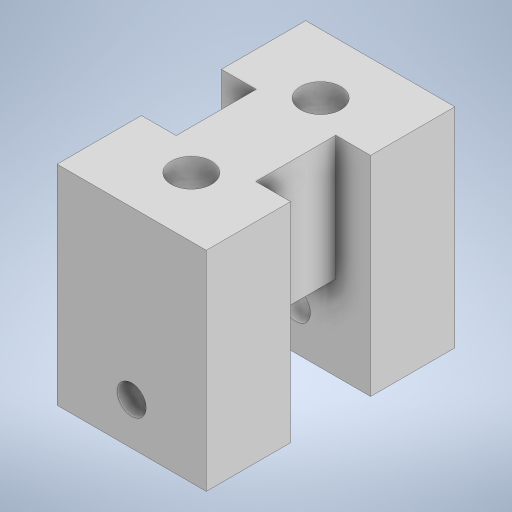
# Autodesk Inventor part: Pièce2
Saved by Autodesk Inventor 2024.1 (Build 281209000, 209)
## iProperties
Created: 2024-04-05
Part Number: Pièce2
Material: Générique
Document SubType Name: Modeling
Designer: chass
Density: 1 g/cm^3
Appearance: Par défaut
Author: chass
Autodesk Inventor part; units mm, degrees
ref_plane "YZ Plane" through (0, 0, 0) normal (1, 0, 0) x (0, 1, 0)
ref_plane "XZ Plane" through (0, 0, 0) normal (0, 1, 0) x (-1, 0, 0)
ref_plane "XY Plane" through (0, 0, 0) normal (0, 0, 1) x (1, 0, 0)
sketch "Esquisse1" plane through (0, 0, 0) normal (0, 1, 0) x (-1, 0, 0)
  line L0 (15, 25) -> (-15, 25)
  line L1 (-15, 25) -> (-15, -25)
  line L2 (-15, -25) -> (15, -25)
  line L3 (15, -25) -> (15, 25)
  line L4 (15, 25) -> (-15, -25)
  line L5 (-15, 25) -> (15, -25)
  circle A0 centre (0, 14) radius 4.05
  line L6 (21, 0) -> (-18, 0)
  circle A1 centre (0, -14) radius 4.05
  point P0 (0, 0)
  point P1 (0, 0)
  point P2 (0, 0)
  dimension "d0" = 50
  dimension "d1" = 30
  dimension "d2" = 8.1
  dimension "d3" = 14
  constraints: 14 end point, 2 centre point, 2 midpoint, 2 parallel, 2 perpendicular, 1 coincident, 1 horizontal, 1 symmetric about line, 1 other
  measures "d0" distance of L2.end L0.start
  measures "d1" distance of L0.start L0.end
  measures "d2" diameter of A0
  measures "d3" distance of point (0, 0) A0.centre
extrude "Extrusion1" add sketch "Esquisse1" along normal blind 10 contours L4 L5 L0 | L3 L6 L4 | L5 L6 L1 | L3 L5 L6 | L5 L2 L4 | L4 L1 L6 | A0 | A1
sketch "Esquisse2" plane through (0, 10, 0) normal (0, 1, 0) x (1, 0, 0)
  circle A0 centre (0, -13) radius 4.05
  line L0 (-17, 0) -> (22, 0)
  circle A1 centre (0, 13) radius 4.05
  line L1 (-15, 25) -> (-15, -25) projected
  line L2 (15, -25) -> (15, 25) projected
  line L3 (-15, -25) -> (15, -25)
  line L4 (15, -25) -> (15, 25)
  line L5 (15, 25) -> (-15, 25)
  line L6 (-15, 25) -> (-15, -25)
  point P0 (0, 0)
  dimension "d6" = 8.1
  dimension "d7" = 13
  constraints: 10 end point, 2 centre point, 2 horizontal, 2 parallel, 1 perpendicular, 1 symmetric about line, 1 other
  measures "d6" diameter of A0
  measures "d7" distance of point (0, 0) A0.centre
extrude "Extrusion2" add sketch "Esquisse2" along normal blind 15
sketch "Esquisse3" plane through (0, 0, 0) normal (0, -1, 0) x (1, 0, 0)
  line L0 (-15, -25) -> (-15, 25) projected
  line L1 (15, 25) -> (15, -25) projected
  line L2 (-15, -8.05) -> (15, -8.05)
  line L3 (15, -8.05) -> (15, 8.05)
  line L4 (15, 8.05) -> (-15, 8.05)
  line L5 (-15, 8.05) -> (-15, -8.05)
  line L6 (-15, -8.05) -> (15, 8.05)
  line L7 (15, -8.05) -> (-15, 8.05)
  line L8 (15, -25) -> (-15, -25) projected
  line L9 (-15, 25) -> (15, 25) projected
  line L10 (-15, -25) -> (15, -25)
  line L11 (15, -25) -> (15, 25)
  line L12 (15, 25) -> (-15, 25)
  line L13 (-15, 25) -> (-15, -25)
  point P0 (0, 0)
  point P1 (0, 0)
  point P2 (0, 0)
  point P3 (-15, 8.05)
  point P4 (15, -8.05)
  dimension "d10" = 16.1
  constraints: 20 end point, 4 parallel, 2 horizontal, 2 midpoint, 2 perpendicular, 2 point on line, 1 coincident
  measures "d10" distance between parallel lines of L4 L2
extrude "Extrusion3" add sketch "Esquisse3" along normal blind 17 contours L0 L2 L1 L8 | L0 L9 L1 L4
sketch "Esquisse4" plane through (-15, 25, 25) normal (0, 0, 1) x (1, 0, 0)
  line L0 (30, -25) -> (30, -42) projected
  line L1 (30, -25) -> (0, -25) projected
  line L2 (30, -42) -> (0, -42)
  line L3 (0, -42) -> (0, -25)
  line L4 (0, -25) -> (30, -25)
  line L5 (30, -25) -> (30, -42)
  circle A0 centre (15, -33.5) radius 2.9
  point P0 (15, -25)
  dimension "d13" = 5.8
  constraints: 8 end point, 2 parallel, 1 centre point, 1 horizontal, 1 perpendicular
  measures "d13" diameter of A0
extrude "Extrusion4" cut sketch "Esquisse4" against normal blind 50 contours A0
sketch "Esquisse5" plane through (0, 0, 0) normal (0, -1, 0) x (1, 0, 0)
  line L0 (15, -8.05) -> (-15, -8.05) projected
  line L1 (-15, 8.05) -> (15, 8.05) projected
  line L2 (-8, -8.05) -> (8, -8.05)
  line L3 (8, -8.05) -> (8, 8.05)
  line L4 (8, 8.05) -> (-8, 8.05)
  line L5 (-8, 8.05) -> (-8, -8.05)
  line L6 (-8, -8.05) -> (8, 8.05)
  line L7 (8, -8.05) -> (-8, 8.05)
  line L8 (-15, -8.05) -> (15, -8.05)
  line L9 (15, -8.05) -> (15, 8.05)
  line L10 (15, 8.05) -> (-15, 8.05)
  line L11 (-15, 8.05) -> (-15, -8.05)
  point P0 (0, 0)
  point P1 (0, 0)
  point P2 (0, 0)
  point P3 (8, -8.05)
  point P4 (-8, 8.05)
  dimension "d16" = 16
  constraints: 20 end point, 4 parallel, 2 horizontal, 2 midpoint, 2 perpendicular, 2 point on line, 1 coincident
  measures "d16" distance between parallel lines of L3 L5
extrude "Extrusion5" cut sketch "Esquisse5" against normal blind 25 contours L0 L3 L1 L9 | L0 L11 L1 L5
